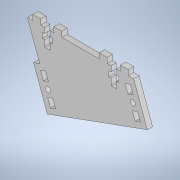
# Autodesk Inventor part: tc_support_front
Saved by Autodesk Inventor 2020.1 (Build 241239000, 239)
## iProperties
Created: 2019-07-16
Part Number: tc_support_front
Material: Acier inoxydable
Document SubType Name: Modeling
Designer: Thibault
Density: 8 g/cm^3
Appearance: Semi-poli
anchor_dist_b: 36.000 mm
anchor_dist_a: 2,000 mm
anchor_dist_top_a: 8.000 mm
tilt_angle: 20,00 deg
tc_plates_dist: 34,000 mm
Author: Thibault
Autodesk Inventor part; units mm, degrees
ref_plane "YZ Plane" through (0, 0, 0) normal (1, 0, 0) x (0, 1, 0)
ref_plane "XZ Plane" through (0, 0, 0) normal (0, 1, 0) x (-1, 0, 0)
ref_plane "XY Plane" through (0, 0, 0) normal (0, 0, 1) x (1, 0, 0)
sketch "Anchor (screw side)" plane through (0, 0, 0) normal (0, 0, 1) x (1, 0, 0)
  circle A0 centre (93.7216, 50.3096) radius 1.05
  line L0 (91.2716, 51.3596) -> (88.1716, 51.3596)
  line L1 (88.1716, 51.3596) -> (88.1716, 49.2596)
  line L2 (88.1716, 49.2596) -> (91.2716, 49.2596)
  line L3 (91.2716, 49.2596) -> (91.2716, 51.3596)
  line L4 (99.2716, 51.3596) -> (96.1716, 51.3596)
  line L5 (96.1716, 51.3596) -> (96.1716, 49.2596)
  line L6 (96.1716, 49.2596) -> (99.2716, 49.2596)
  line L7 (99.2716, 49.2596) -> (99.2716, 51.3596)
  line L8 (91.2716, 51.3596) -> (96.1716, 49.2596) construction
  line L9 (96.1716, 51.3596) -> (91.2716, 49.2596) construction
  line L10 (86.1716, 53.3596) -> (101.2716, 53.3596) construction
  line L11 (101.2716, 53.3596) -> (101.2716, 47.2596) construction
  line L12 (101.2716, 47.2596) -> (86.1716, 47.2596) construction
  line L13 (86.1716, 47.2596) -> (86.1716, 53.3596) construction
  point P0 (103.5798, 50.1132)
  dimension "d27" = 2.1
  dimension "d28" = 3.1
  dimension "d29" = 2.1
  dimension "d32" = 4.9
  dimension "d34" = 2
  dimension "d35_1" = 2
  dimension "d36_1" = 2
  dimension "d37" = 2
  measures "d27" diameter of A0
  measures "d28" distance of L2.end L1.end
  measures "d29" distance of L1.end L0.end
  measures "d32" distance between parallel lines of L5 L3
  measures "d34" distance between parallel lines of L0 L10
  measures "d35_1" distance between parallel lines of L12 L2
  measures "d36_1" distance between parallel lines of L11 L7
  measures "d37" distance between parallel lines of L13 L1
sketch "Anchor (nut side)" plane through (0, 0, 0) normal (0, 0, 1) x (1, 0, 0)
  line L0 (10, 0) -> (8.55, 0)
  line L1 (8.55, 0) -> (8.55, -2)
  line L2 (8.55, -2) -> (9.35, -2)
  line L3 (9.35, -2) -> (9.35, -4)
  line L4 (5.65, -4) -> (5.65, -2)
  line L5 (5.65, -2) -> (6.45, -2)
  line L6 (6.45, -2) -> (6.45, 0)
  line L7 (6.45, 0) -> (5, 0)
  line L8 (2, 0) -> (2, 2)
  line L9 (2, 0) -> (3, 0) construction
  line L10 (2, 2) -> (5, 2)
  line L11 (5, 2) -> (5, 0)
  line L12 (10, 0) -> (10, 2)
  line L13 (10, 2) -> (13, 2)
  line L14 (13, 2) -> (13, 0)
  line L15 (0, 0) -> (2, 0)
  line L16 (13, 0) -> (15, 0)
  line L17 (5.65, -4) -> (6.45, -4)
  line L18 (9.35, -4) -> (8.55, -4)
  line L19 (6.45, -4) -> (6.45, -6.25)
  line L20 (8.55, -4) -> (8.55, -6.25)
  line L21 (6.7, -6.5) -> (7.5, -6.5)
  arc A0 (6.45, -6.25) -> (6.7, -6.5) centre (6.7, -6.25) ccw
  arc A1 (8.3, -6.5) -> (8.55, -6.25) centre (8.3, -6.25) ccw
  line L22 (7.5, -6.5) -> (8.3, -6.5)
  line L23 (7.5, -3.8983) -> (7.5, -9.959) construction
  point P0 (9.1321, -0.6227)
  point P1 (6.45, -6.5)
  point P2 (8.55, -6.5)
  dimension "d3" = 2
  dimension "d7" = 5
  dimension "d10" = 1.45
  dimension "d11" = 2
  dimension "d12" = 0.8
  dimension "d13" = 2
  dimension "d14" = 0.8
  dimension "d15" = 2.1
  dimension "d18" = 2
  dimension "d19" = 0.8
  dimension "d20" = 0.8
  dimension "d21" = 2.5
  dimension "d22" = 2.5
  dimension "d23" = 2.1
  dimension "d38" = 2
  dimension "d39" = 0.25
  dimension "d120" = 3
  measures "d3" distance of L15.start L8.start
  measures "d7" distance of L7.end L0.start
  measures "d10" distance of L0.start L0.end
  measures "d11" distance of L0.end L1.end
  measures "d12" distance of L1.end L2.end
  measures "d13" distance of L2.end L3.end
  measures "d14" distance of L4.end L5.end
  measures "d15" distance of L6.end L0.end
  measures "d18" distance of L14.end L16.end
  measures "d19" distance of L4.start L17.end
  measures "d20" distance of L3.end L18.end
  measures "d21" distance of L17.end point (6.45, -6.5)
  measures "d22" distance of L18.end point (8.55, -6.5)
  measures "d23" distance of L17.end L18.end
  measures "d38" distance between parallel lines of L15 L10
  measures "d39" radius of A0
  measures "d120" distance of L8.end L10.end
derived "shared_parameters.ipt"
sketch "Esquisse1" plane through (0, 0, 0) normal (0, 0, 1) x (1, 0, 0)
  line L0 (82.6044, -30.9853) -> (77.4901, -16.9338)
  line L1 (82.6044, -30.9853) -> (47.2394, -43.8571)
  line L2 (-2.0657, -1.8526) -> (7.9343, -1.7975) construction
  line L3 (42.0749, -29.6677) -> (37.4401, -16.9338)
  line L4 (52.4401, -16.9338) -> (62.4901, -16.9338)
  line L5 (39.7582, -30.5109) -> (44.9227, -44.7003)
  line L6 (39.7582, -30.5109) -> (42.0749, -29.6677)
  line L7 (47.2394, -43.8571) -> (47.2394, -43.8571)
  line L8 (44.9227, -44.7003) -> (47.2394, -43.8571)
  circle A0 centre (77.1561, -24.9338) radius 1.05
  line L9 (77.0074, -27.5951) -> (78.0676, -30.5082)
  line L10 (78.0676, -30.5082) -> (80.041, -29.7899)
  line L11 (80.041, -29.7899) -> (78.9807, -26.8769)
  line L12 (78.9807, -26.8769) -> (77.0074, -27.5951)
  line L13 (74.2712, -20.0776) -> (75.3315, -22.9906)
  line L14 (75.3315, -22.9906) -> (77.3048, -22.2724)
  line L15 (77.3048, -22.2724) -> (76.2446, -19.3593)
  line L16 (76.2446, -19.3593) -> (74.2712, -20.0776)
  line L17 (77.0074, -27.5951) -> (77.3048, -22.2724) construction
  line L18 (75.3315, -22.9906) -> (78.9807, -26.8769) construction
  line L19 (76.8723, -33.0716) -> (71.7078, -18.8822) construction
  line L20 (71.7078, -18.8822) -> (77.4399, -16.7959) construction
  line L21 (77.4399, -16.7959) -> (82.6044, -30.9853) construction
  line L22 (82.6044, -30.9853) -> (76.8723, -33.0716) construction
  circle A1 centre (45.2065, -36.5624) radius 1.05
  line L23 (45.3553, -33.9011) -> (44.295, -30.988)
  line L24 (44.295, -30.988) -> (42.3216, -31.7063)
  line L25 (42.3216, -31.7063) -> (43.3819, -34.6193)
  line L26 (43.3819, -34.6193) -> (45.3553, -33.9011)
  line L27 (48.0914, -41.4186) -> (47.0312, -38.5056)
  line L28 (47.0312, -38.5056) -> (45.0578, -39.2238)
  line L29 (45.0578, -39.2238) -> (46.1181, -42.1369)
  line L30 (46.1181, -42.1369) -> (48.0914, -41.4186)
  line L31 (45.3553, -33.9011) -> (45.0578, -39.2238) construction
  line L32 (47.0312, -38.5056) -> (43.3819, -34.6193) construction
  line L33 (45.4903, -28.4246) -> (50.6549, -42.614) construction
  line L34 (50.6549, -42.614) -> (44.9227, -44.7003) construction
  line L35 (44.9227, -44.7003) -> (39.7582, -30.5109) construction
  line L36 (39.7582, -30.5109) -> (45.4903, -28.4246) construction
  line L37 (47.4401, -16.9338) -> (45.9901, -16.9338)
  line L38 (45.9901, -16.9338) -> (45.9901, -18.9338)
  line L39 (45.9901, -18.9338) -> (46.7901, -18.9338)
  line L40 (46.7901, -18.9338) -> (46.7901, -20.9338)
  line L41 (43.0901, -20.9338) -> (43.0901, -18.9338)
  line L42 (43.0901, -18.9338) -> (43.8901, -18.9338)
  line L43 (43.8901, -18.9338) -> (43.8901, -16.9338)
  line L44 (43.8901, -16.9338) -> (42.4401, -16.9338)
  line L45 (39.4401, -16.9338) -> (39.4401, -14.9338)
  line L46 (39.4401, -16.9338) -> (40.4401, -16.9338) construction
  line L47 (39.4401, -14.9338) -> (42.4401, -14.9338)
  line L48 (42.4401, -14.9338) -> (42.4401, -16.9338)
  line L49 (47.4401, -16.9338) -> (47.4401, -14.9338)
  line L50 (47.4401, -14.9338) -> (50.4401, -14.9338)
  line L51 (50.4401, -14.9338) -> (50.4401, -16.9338)
  line L52 (37.4401, -16.9338) -> (39.4401, -16.9338)
  line L53 (50.4401, -16.9338) -> (52.4401, -16.9338)
  line L54 (43.0901, -20.9338) -> (43.8901, -20.9338)
  line L55 (46.7901, -20.9338) -> (45.9901, -20.9338)
  line L56 (43.8901, -20.9338) -> (43.8901, -23.1838)
  line L57 (45.9901, -20.9338) -> (45.9901, -23.1838)
  line L58 (44.1401, -23.4338) -> (44.9401, -23.4338)
  arc A2 (43.8901, -23.1838) -> (44.1401, -23.4338) centre (44.1401, -23.1838) ccw
  arc A3 (45.7401, -23.4338) -> (45.9901, -23.1838) centre (45.7401, -23.1838) ccw
  line L59 (44.9401, -23.4338) -> (45.7401, -23.4338)
  line L60 (44.9401, -20.832) -> (44.9401, -26.8928) construction
  line L61 (72.4901, -16.9338) -> (71.0401, -16.9338)
  line L62 (71.0401, -16.9338) -> (71.0401, -18.9338)
  line L63 (71.0401, -18.9338) -> (71.8401, -18.9338)
  line L64 (71.8401, -18.9338) -> (71.8401, -20.9338)
  line L65 (68.1401, -20.9338) -> (68.1401, -18.9338)
  line L66 (68.1401, -18.9338) -> (68.9401, -18.9338)
  line L67 (68.9401, -18.9338) -> (68.9401, -16.9338)
  line L68 (68.9401, -16.9338) -> (67.4901, -16.9338)
  line L69 (64.4901, -16.9338) -> (64.4901, -14.9338)
  line L70 (64.4901, -16.9338) -> (65.4901, -16.9338) construction
  line L71 (64.4901, -14.9338) -> (67.4901, -14.9338)
  line L72 (67.4901, -14.9338) -> (67.4901, -16.9338)
  line L73 (72.4901, -16.9338) -> (72.4901, -14.9338)
  line L74 (72.4901, -14.9338) -> (75.4901, -14.9338)
  line L75 (75.4901, -14.9338) -> (75.4901, -16.9338)
  line L76 (62.4901, -16.9338) -> (64.4901, -16.9338)
  line L77 (75.4901, -16.9338) -> (77.4901, -16.9338)
  line L78 (68.1401, -20.9338) -> (68.9401, -20.9338)
  line L79 (71.8401, -20.9338) -> (71.0401, -20.9338)
  line L80 (68.9401, -20.9338) -> (68.9401, -23.1838)
  line L81 (71.0401, -20.9338) -> (71.0401, -23.1838)
  line L82 (69.1901, -23.4338) -> (69.9901, -23.4338)
  arc A4 (68.9401, -23.1838) -> (69.1901, -23.4338) centre (69.1901, -23.1838) ccw
  arc A5 (70.7901, -23.4338) -> (71.0401, -23.1838) centre (70.7901, -23.1838) ccw
  line L83 (69.9901, -23.4338) -> (70.7901, -23.4338)
  line L84 (69.9901, -20.832) -> (69.9901, -26.8928) construction
  point P0 (77.1561, -24.9338)
  point P1 (77.4901, -16.9338)
  dimension "d44" = 2
  dimension "d45" = 0.4653
  dimension "d55" = 40.05
  dimension "tc_plates_dist" = 34
  constraints: 18 end point, 3 horizontal, 2 perpendicular, 2 point on line, 1 collinear, 1 parallel, 14 other
  measures "d55" distance of L3.end L0.end
  measures "tc_plates_dist" distance of point (45.207, -36.562) point (77.156, -24.934)
extrude "Extrusion1" add sketch "Esquisse1" along normal blind 2
equation "\"d55\" = tc_base_back_width"
equation "\"d35\" = sheet_thickness"
equation "\"tc_base_back_width\" = 40.05"
equation "\"sheet_thickness\" = 2"
